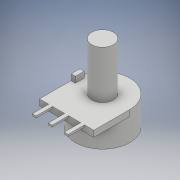
# Autodesk Inventor part: potentiometer
Saved by Autodesk Inventor 2018 (Build 220112000, 112)
## iProperties
Created: 2017-12-11
Part Number: potentiometer
Material: Generic
Document SubType Name: Modeling
Designer: caleb
Density: 1 g/cm^3
Appearance: Default
Author: caleb
Autodesk Inventor part; units mm, degrees
ref_plane "YZ Plane" through (0, 0, 0) normal (1, 0, 0) x (0, 1, 0)
ref_plane "XZ Plane" through (0, 0, 0) normal (0, 1, 0) x (-1, 0, 0)
ref_plane "XY Plane" through (0, 0, 0) normal (0, 0, 1) x (1, 0, 0)
sketch "Sketch1" plane through (0, 0, 0) normal (0, 0, 1) x (1, 0, 0)
  circle A0 centre (0, 0) radius 3.429
  circle A1 centre (0, 0) radius 8.636
  line L0 (-8.636, 0) -> (-8.636, -11.43)
  line L1 (-8.636, -11.43) -> (8.636, -11.43)
  line L2 (8.636, -11.43) -> (8.636, 0)
  point P0 (0, 8.636)
  dimension "d0" = 6.858
  dimension "d1" = 17.272
  dimension "d2" = 20.066
  constraints: 6 end point, 3 point on circle, 2 centre point, 2 coincident, 2 horizontal alignment, 2 vertical, 1 perpendicular, 1 vertical alignment
  measures "d0" diameter of A0
  measures "d1" diameter of A1
  measures "d2" distance from line of L1 point (0, 8.636)
extrude "Extrusion1" add sketch "Sketch1" against normal blind 9.144 contours A0 | A1
extrude "Extrusion2" add sketch "Sketch1" along normal blind 15.24 contours A0
extrude "Extrusion3" add sketch "Sketch1" against normal blind 1.9558 contours L2 L1 L0 A1
sketch "Sketch2" plane through (0, 0, 0) normal (0, 0, 1) x (1, 0, 0)
  circle A0 centre (0, 0) radius 3.429 construction
  arc A1 (8.636, 0) -> (-8.636, 0) centre (0, 0) ccw construction
  line L0 (-8.636, 0) -> (-8.636, -11.43) construction
  line L1 (-8.636, -11.43) -> (8.636, -11.43) construction
  line L2 (8.636, -11.43) -> (8.636, 0) construction
  circle A2 centre (0, 0) radius 8.636 construction
  line L3 (-8.5223, -1.397) -> (-7.239, -1.397)
  line L4 (-7.239, -1.397) -> (-7.239, 1.397)
  line L5 (-7.239, 1.397) -> (-8.5223, 1.397)
  arc A3 (8.636, 0) -> (-8.5223, 1.397) centre (0, 0) ccw construction
  arc A4 (-8.5223, -1.397) -> (8.636, 0) centre (0, 0) ccw
  arc A5 (-8.5223, 1.397) -> (-8.5223, -1.397) centre (0, 0) ccw
  point P0 (-7.239, 0)
  dimension "d9" = 2.794
  dimension "d10" = 1.397
  constraints: 8 point on circle, 7 end point, 3 centre point, 2 perpendicular, 1 coincident, 1 concentric, 1 horizontal, 1 horizontal alignment, 1 midpoint
  measures "d9" distance of L3.end L4.end
  measures "d10" distance from line of L3.end L0
extrude "Extrusion4" add sketch "Sketch2" along normal blind 1.905
sketch "Sketch3" plane through (0, 0, 0) normal (0, 0, 1) x (1, 0, 0)
  line L0 (-8.5223, 1.397) -> (-7.239, 1.397) projected
  line L1 (-7.239, 1.397) -> (-7.239, -1.397) projected
  line L2 (-7.239, -1.397) -> (-8.5223, -1.397) projected
  arc A0 (-8.636, 0) -> (-8.5223, -1.397) centre (0, 0) ccw projected
  line L3 (-8.636, 0) -> (-8.636, -11.43) projected
  line L4 (-8.636, -11.43) -> (8.636, -11.43) projected
  line L5 (8.636, -11.43) -> (8.636, 0) projected
  arc A1 (8.636, 0) -> (-8.5223, 1.397) centre (0, 0) ccw projected
  circle A2 centre (0, 0) radius 3.429 projected
  line L6 (-8.636, -11.43) -> (8.636, -11.43) projected
  line L7 (-5.68, -11.43) -> (-4.48, -11.43)
  line L8 (-4.48, -11.43) -> (-4.48, -16.63)
  line L9 (-4.48, -16.63) -> (-5.68, -16.63)
  line L10 (-5.68, -16.63) -> (-5.68, -11.43)
  line L11 (-0.6, -11.43) -> (0.6, -11.43)
  line L12 (0.6, -11.43) -> (0.6, -16.63)
  line L13 (0.6, -16.63) -> (-0.6, -16.63)
  line L14 (-0.6, -16.63) -> (-0.6, -11.43)
  line L15 (4.48, -11.43) -> (5.68, -11.43)
  line L16 (5.68, -11.43) -> (5.68, -16.63)
  line L17 (5.68, -16.63) -> (4.48, -16.63)
  line L18 (4.48, -16.63) -> (4.48, -11.43)
  point P0 (0, -16.63)
  point P1 (0, -11.43)
  dimension "d13" = 5.08
  dimension "d14" = 5.08
  dimension "d15" = 5.2
  dimension "d16" = 1.2
  constraints: 24 end point, 6 parallel, 4 point on line, 3 equal length, 3 horizontal, 3 perpendicular, 2 midpoint, 1 vertical alignment
  measures "d13" distance of L9.end L13.end
  measures "d14" distance of L16.end L12.end
  measures "d15" distance of L9.end L7.start
  measures "d16" distance of L16.end L17.end
extrude "Extrusion5" add sketch "Sketch3" against normal blind 0.6 contours L16 L17 L18 L4 | L12 L13 L14 L4 | L4 L8 L9 L10
body "Solid1"
